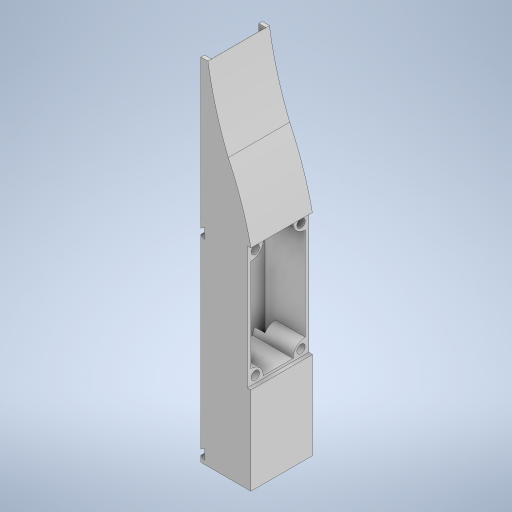
# Autodesk Inventor part: case_ver4
Saved by Autodesk Inventor 2024 (Build 280153000, 153)
## iProperties
Created: 2023-11-10
Part Number: case_ver4
Material: 一般
Document SubType Name: Modeling
Designer: Kota Taga
Density: 1 g/cm^3
Appearance: 既定
Author: Kota Taga
## iProperties of the stored document case_3D プリント.ipt
Created: 2023-11-10
Part Number: case_3D プリント
Material: 一般
Document SubType Name: Modeling
Designer: Kota Taga
Density: 1 g/cm^3
Appearance: 既定
Author: Kota Taga
Autodesk Inventor part; units mm, degrees
ref_plane "YZ Plane" through (0, 0, 0) normal (1, 0, 0) x (0, 1, 0)
ref_plane "XZ Plane" through (0, 0, 0) normal (0, 1, 0) x (-1, 0, 0)
ref_plane "XY Plane" through (0, 0, 0) normal (0, 0, 1) x (1, 0, 0)
sketch "スケッチ1" plane through (0, 0, 0) normal (0, 1, 0) x (-1, 0, 0)
  line L0 (10.25, 18.25) -> (-10.25, 18.25)
  line L1 (-10.25, 18.25) -> (-10.25, -18.25)
  line L2 (-10.25, -18.25) -> (10.25, -18.25)
  line L3 (10.25, -18.25) -> (10.25, 18.25)
  line L4 (23.2518, 0) -> (-17.5836, 0) projected
  line L5 (0, -27.65) -> (0, 27.65) projected
  line L6 (11.75, 19.75) -> (-11.75, 19.75)
  line L7 (-11.75, 19.75) -> (-11.75, -19.75)
  line L8 (-11.75, -19.75) -> (11.75, -19.75)
  line L9 (11.75, -19.75) -> (11.75, 19.75)
  line L10 (17.4182, 0.0611) -> (-9.1818, 0.0611)
  point P0 (0, 0)
  dimension "d0" = 36.5
  dimension "d1" = 20.5
  dimension "d2" = 1.5
  constraints: 18 end point, 5 parallel, 2 perpendicular, 1 horizontal, 5 other
  measures "d0" distance of L2.end L0.start
  measures "d1" distance of L0.start L0.end
  measures "d2" distance between parallel lines of L3 L9
extrude "押し出し1" add sketch "スケッチ1" along normal blind 70 contours L0 L5 L6 L9 L10 L3 | L0 L1 L4 L7 L6 L5 | L10 L9 L4 L3 | L4 L9 L8 L5 L2 L3 | L1 L2 L5 L8 L7 L4
sketch "スケッチ2" plane through (-11.75, 0, -19.75) normal (-1, 0, 0) x (0, 0, 1)
  line L0 (38, 0) -> (1.5, 0) projected
  line L1 (0, 70) -> (1.75, 70)
  line L2 (1.75, 70) -> (1.75, 0)
  line L3 (1.75, 0) -> (0, 0)
  line L4 (0, 0) -> (0, 70)
  line L5 (39.5, 0) -> (39.5, 70) projected
  line L6 (39.5, 70) -> (37.75, 70)
  line L7 (37.75, 70) -> (37.75, 0)
  line L8 (37.75, 0) -> (39.5, 0)
  line L9 (39.5, 0) -> (39.5, 70)
  point P0 (19.75, 0)
  point P1 (1.5, 0)
  dimension "d5" = 1.75
  dimension "d6" = 1.75
  constraints: 16 end point, 4 parallel, 2 horizontal, 2 perpendicular, 2 point on line
  measures "d5" distance of L2.end L3.end
  measures "d6" distance of L8.end L7.end
extrude "押し出し2" add sketch "スケッチ2" along normal blind 19
sketch "スケッチ3" plane through (11.75, 0, 19.75) normal (1, 0, 0) x (0, 0, -1)
  line L0 (0, 70) -> (39.5, 70) projected
  line L1 (39.5, 0) -> (39.5, 70) projected
  line L2 (0, 70) -> (39.5, 70)
  line L3 (39.5, 70) -> (39.5, 0)
  line L4 (39.5, 0) -> (0, 0)
  line L5 (0, 0) -> (0, 70)
  point P0 (19.75, 0)
  constraints: 8 end point, 2 parallel, 1 horizontal, 1 perpendicular
extrude "押し出し3" cut sketch "スケッチ3" against normal up to surface (1.5 mm away)
sketch "スケッチ4" plane through (10.25, 0, 18.25) normal (1, 0, 0) x (0, 0, -1)
  line L0 (-1.5, 70) -> (0, 70) projected
  line L1 (0, 0) -> (0, 70) projected
  line L2 (-1.5, 70) -> (0, 70)
  line L3 (0, 70) -> (0, 0)
  line L4 (0, 0) -> (-1.5, 0)
  line L5 (-1.5, 0) -> (-1.5, 70)
  line L6 (38, 70) -> (38, 0) projected
  line L7 (36.5, 0) -> (36.5, 70) projected
  line L8 (38, 70) -> (36.5, 70)
  line L9 (36.5, 70) -> (36.5, 0)
  line L10 (36.5, 0) -> (38, 0)
  line L11 (38, 0) -> (38, 70)
  point P0 (18.25, 0)
  constraints: 16 end point, 4 parallel, 2 horizontal, 2 perpendicular
extrude "押し出し4" add sketch "スケッチ4" along normal blind 14.5
sketch "スケッチ5" plane through (-10.25, 0, 18.25) normal (1, 0, 0) x (0, 0, -1)
  line L0 (38, 70) -> (36.5, 70) projected
  line L1 (0, 0) -> (0, 70) projected
  line L2 (36.5, 70) -> (0, 70)
  line L3 (0, 70) -> (0, 68.5)
  line L4 (0, 68.5) -> (36.5, 68.5)
  line L5 (36.5, 68.5) -> (36.5, 70)
  line L6 (0.25, 0) -> (0.25, 70) projected
  line L7 (36.5, 0) -> (36.5, 70) projected
  line L8 (0.25, 0) -> (36.5, 0)
  line L9 (36.5, 0) -> (36.5, 1.5)
  line L10 (36.5, 1.5) -> (0.25, 1.5)
  line L11 (0.25, 1.5) -> (0.25, 0)
  point P0 (18.25, 0)
  point P1 (0.25, 1.5)
  dimension "d13" = 1.5
  dimension "d14" = 1.5
  constraints: 16 end point, 4 parallel, 2 horizontal, 2 perpendicular, 2 point on line
  measures "d13" distance between parallel lines of L2 L4
  measures "d14" distance of L9.end L8.end
extrude "押し出し5" add sketch "スケッチ5" along normal up to surface (35 mm away) contours L1 L2 L6 L4 | L6 L2 L5 L4 | L10 L7 L8 L6
sketch "スケッチ6" plane through (0, 70, 0) normal (0, 1, 0) x (1, 0, 0)
  line L0 (24.75, -18) -> (24.75, 18.25) projected
  line L1 (24.75, -10) -> (14.75, -10)
  line L2 (14.75, -10) -> (14.75, 10)
  line L3 (14.75, 10) -> (24.75, 10)
  line L4 (24.75, 10) -> (24.75, -10)
  line L5 (-41.85, 0) -> (35.85, 0) projected
  line L6 (0, 27.65) -> (0, -27.65) projected
  point P0 (0, 0)
  dimension "d17" = 10
  dimension "d18" = 20
  constraints: 8 end point, 2 parallel, 1 horizontal, 1 perpendicular, 1 point on line, 1 other
  measures "d17" distance of L2.end L3.end
  measures "d18" distance of L1.end L2.end
extrude "押し出し6" cut sketch "スケッチ6" against normal up to surface (70 mm away)
sketch "スケッチ7" plane through (0, 0, 0) normal (0, -1, 0) x (1, 0, 0)
  line L0 (-10.25, 18.25) -> (-10.25, 18) projected
  line L1 (-10.25, 18) -> (24.75, 18) projected
  line L2 (-10.25, 18.25) -> (24.75, 18.25)
  line L3 (24.75, 18.25) -> (24.75, 18)
  line L4 (24.75, 18) -> (-10.25, 18)
  line L5 (-10.25, 18) -> (-10.25, 18.25)
  point P0 (0, 0)
  constraints: 8 end point, 2 parallel, 1 horizontal, 1 perpendicular
extrude "押し出し7" add sketch "スケッチ7" against normal up to surface (1.5 mm away)
sketch "スケッチ8" plane through (-10.25, 1.5, -18.25) normal (1, 0, 0) x (0, 0, -1)
  line L0 (0, 67) -> (-36.5, 67) projected
  circle A0 centre (-36.5, 67) radius 7.5
  line L1 (0, 67) -> (0, 0) projected
  circle A1 centre (0, 67) radius 7.5
  line L2 (-8.25, 0) -> (0, 0) projected
  circle A2 centre (0, 0) radius 7.5
  line L3 (-36.5, 0) -> (-36.5, 67) projected
  circle A3 centre (-36.5, 0) radius 7.5
  line L4 (-36.5, 7.5) -> (-36.5, 0)
  line L5 (-28.25, 0) -> (-36.5, 0) projected
  line L6 (-29, 0) -> (-36.5, 0)
  point P0 (-18.25, -1.5)
  point P1 (-36.5, 59.5)
  point P2 (-29, 67)
  point P3 (-7.5, 67)
  point P4 (0, 59.5)
  point P5 (0, 7.5)
  point P6 (-7.5, 0)
  dimension "d23" = 15
  dimension "d24" = 15
  dimension "d25" = 15
  dimension "d26" = 15
  constraints: 4 centre point, 4 end point, 2 coincident, 2 point on circle, 2 point on line, 1 collinear, 1 vertical
  measures "d23" diameter of A0
  measures "d24" diameter of A1
  measures "d25" diameter of A2
  measures "d26" diameter of A3
extrude "押し出し8" add sketch "スケッチ8" along normal up to surface (35 mm away) contours A0 L3 L0 | L1 A1 L0 | L1 L2 A2 | L3 A3 L5 picked at (-31.5627, 66.4437) picked at (-4.9373, 66.4437) picked at (-3.5133, 3.5133) picked at (-33.8566, 4.207)
sketch "スケッチ9" plane through (24.75, 0, 18.25) normal (1, 0, 0) x (0, 0, -1)
  circle A0 centre (2.5, 66) radius 2.4
  line L0 (-1.5, 70) -> (-1.5, 0) projected
  line L1 (8.25, 70) -> (-1.5, 70) projected
  circle A1 centre (34, 66) radius 2.4
  circle A2 centre (34, 4) radius 2.4
  circle A3 centre (2.5, 4) radius 2.4
  line L2 (8.25, 0) -> (-1.5, 0) projected
  line L3 (38, 0) -> (38, 70) projected
  line L4 (38, 0) -> (28.25, 0) projected
  line L5 (38, 70) -> (28.25, 70) projected
  point P0 (18.25, 0)
  point P1 (33.125, 0)
  dimension "d29" = 4.8
  dimension "d30" = 4
  dimension "d31" = 4
  dimension "d32" = 4
  dimension "d33" = 4
  dimension "d34" = 4.8
  dimension "d35" = 4
  dimension "d36" = 4
  dimension "d37" = 4.8
  dimension "d38" = 4
  dimension "d39" = 4
  dimension "d40" = 4.8
  constraints: 4 centre point, 1 midpoint
  measures "d29" diameter of A0
  measures "d30" distance from line of L0 A0.centre
  measures "d31" distance from line of L1 A0.centre
  measures "d32" distance from line of L2 A3.centre
  measures "d33" distance from line of L0 A3.centre
  measures "d34" diameter of A3
  measures "d35" distance from line of L3 A2.centre
  measures "d36" vertical distance of point (33.125, 0) A2.centre
  measures "d37" diameter of A2
  measures "d38" distance from line of L5 A1.centre
  measures "d39" distance from line of L3 A1.centre
  measures "d40" diameter of A1
extrude "押し出し9" cut sketch "スケッチ9" against normal blind 5
sketch "スケッチ10" plane through (0, 0, 0) normal (0, -1, 0) x (1, 0, 0)
  line L0 (14.75, 10) -> (24.75, 10) projected
  line L1 (24.75, -10) -> (14.75, -10) projected
  line L2 (24.75, 10) -> (14.75, 10)
  line L3 (14.75, 10) -> (14.75, -10)
  line L4 (14.75, -10) -> (24.75, -10)
  line L5 (24.75, -10) -> (24.75, 10)
  circle A0 centre (24.75, 0) radius 4
  point P0 (0, 0)
  point P1 (24.75, -4)
  point P2 (24.75, 4)
  dimension "d43" = 8
  constraints: 8 end point, 2 parallel, 1 centre point, 1 horizontal, 1 midpoint, 1 perpendicular
  measures "d43" diameter of A0
extrude "押し出し10" add sketch "スケッチ10" against normal up to surface (1.5 mm away) contours L0 L5 A0 L1 L3
sketch "スケッチ11" plane through (24.75, 0, 18.25) normal (1, 0, 0) x (0, 0, -1)
  line L0 (-1.5, 70) -> (-1.5, 0) projected
  line L1 (38, 0) -> (38, 70) projected
  line L2 (-1.5, 70) -> (38, 70)
  line L3 (38, 70) -> (38, 0)
  line L4 (38, 0) -> (-1.5, 0)
  line L5 (-1.5, 0) -> (-1.5, 70)
  point P0 (18.25, 0)
  point P1 (-1.5, 0)
  constraints: 8 end point, 2 parallel, 1 horizontal, 1 perpendicular
extrude "押し出し11" cut sketch "スケッチ11" against normal blind 10
sketch "スケッチ13" plane through (-30.75, 0, -19.75) normal (0, 0, -1) x (-1, 0, 0)
  arc A0 (-33.4976, 96.3635) -> (-19, 122.148) centre (-76.3491, 137.4253) ccw projected
  line L0 (-19, 122.148) -> (-22.9342, 122.148)
  line L1 (-22.9342, 122.148) -> (-22.9342, 137.4253)
  line L2 (-22.9342, 137.4253) -> (-19, 137.4253)
  line L3 (-19, 137.4253) -> (-19, 122.148)
  point P0 (-30.75, 0)
  constraints: 8 end point, 2 parallel, 1 horizontal, 1 perpendicular
extrude "押し出し13" cut sketch "スケッチ13" against normal up to surface (39.5 mm away)
sketch "スケッチ14" plane through (-30.75, 0, 19.75) normal (0, 0, 1) x (1, 0, 0)
  arc A0 (19, 122.148) -> (33.4976, 96.3635) centre (76.3491, 137.4253) ccw projected
  line L0 (19, 122.148) -> (19, 70)
  line L1 (45.5, 70) -> (0, 70) projected
  line L2 (19, 70) -> (43.4941, 70)
  arc A1 (43.4941, 70) -> (33.4976, 96.3635) centre (-6.67, 66.0559) ccw projected
  arc A2 (43.4941, 70) -> (33.4976, 96.3635) centre (-6.67, 66.0559) ccw
  arc A3 (19, 122.148) -> (33.4976, 96.3635) centre (76.3491, 137.4253) ccw
  point P0 (30.75, 0)
  constraints: 4 end point, 4 point on circle, 2 centre point, 2 concentric, 1 horizontal, 1 point on line, 1 vertical
extrude "押し出し14" add sketch "スケッチ14" against normal blind 2
mirror "ミラー1" about plane through (0, 0, 0) normal (0, 0, 1) of "押し出し14"
sketch "スケッチ15" plane through (0, 70, 0) normal (0, 1, 0) x (1, 0, 0)
  line L0 (-11.75, 17.75) -> (-11.75, -17.75) projected
  line L1 (12.7441, 17.75) -> (-11.75, 17.75) projected
  line L2 (-11.75, -17.75) -> (0.497, -17.75)
  line L3 (0.497, -17.75) -> (0.497, 17.75)
  line L4 (0.497, 17.75) -> (-11.75, 17.75)
  line L5 (-11.75, 17.75) -> (-11.75, -17.75)
  point P0 (0, 0)
  constraints: 8 end point, 2 parallel, 1 horizontal, 1 midpoint, 1 perpendicular
extrude "押し出し15" cut sketch "スケッチ15" against normal blind 2
sketch "スケッチ17" plane through (0, 70, 0) normal (0, 1, 0) x (1, 0, 0)
  line L0 (-30.75, -19.75) -> (-30.75, -18) projected
  line L1 (-11.75, -18) -> (-30.75, -18) projected
  line L2 (-30.75, -19.75) -> (-11.75, -19.75)
  line L3 (-11.75, -19.75) -> (-11.75, -18)
  line L4 (-11.75, -18) -> (-30.75, -18)
  line L5 (-30.75, -18) -> (-30.75, -19.75)
  line L6 (-11.75, 19.75) -> (-30.75, 19.75) projected
  line L7 (-11.75, 18) -> (-30.75, 18) projected
  line L8 (-30.75, 19.75) -> (-11.75, 19.75)
  line L9 (-11.75, 19.75) -> (-11.75, 18)
  line L10 (-11.75, 18) -> (-30.75, 18)
  line L11 (-30.75, 18) -> (-30.75, 19.75)
  point P0 (0, 0)
  constraints: 16 end point, 4 parallel, 2 horizontal, 2 perpendicular
extrude "押し出し17" [suppressed]
sketch "スケッチ18" plane through (-30.75, 0, 19.75) normal (0, 0, 1) x (1, 0, 0)
  line L0 (0, 0) -> (0, 122.148) projected
  line L1 (45.5, 0) -> (45.5, 70) projected
  line L2 (0, 0) -> (45.5, 0)
  line L3 (45.5, 0) -> (45.5, 70)
  line L4 (45.5, 70) -> (0, 70)
  line L5 (0, 70) -> (0, 0)
  line L6 (0, 70) -> (0, 122.148)
  line L7 (19, 68) -> (19, 122.148) projected
  line L8 (0, 122.148) -> (21.0723, 122.148) projected
  line L9 (0, 122.148) -> (19.5705, 122.148)
  arc A0 (21.4839, 120.7302) -> (19.5705, 122.148) centre (19.5705, 120.148) ccw projected
  arc A1 (21.4839, 120.7302) -> (19.5705, 122.148) centre (19.5705, 120.148) ccw
  arc A2 (45.5, 70) -> (35.0218, 97.6639) centre (-6.67, 66.0559) ccw projected
  arc A3 (21.4839, 120.7302) -> (35.0218, 97.6639) centre (76.3491, 137.4253) ccw
  arc A4 (45.5, 70) -> (35.0218, 97.6639) centre (-6.67, 66.0559) ccw
  point P0 (30.75, 0)
  constraints: 12 end point, 6 point on circle, 3 centre point, 3 parallel, 2 tangent, 1 collinear, 1 horizontal, 1 perpendicular
extrude "押し出し18" add sketch "スケッチ18" along normal blind 1
sketch "スケッチ19" plane through (14.75, 0, -19.75) normal (0, 0, -1) x (-1, 0, 0)
  arc A0 (10.4782, 97.6639) -> (0, 70) centre (52.17, 66.0559) ccw projected
  line L0 (45.5, 122.148) -> (45.5, 0) projected
  line L1 (0, 70) -> (45.5, 70)
  line L2 (45.5, 70) -> (45.5, 0)
  line L3 (45.5, 0) -> (0, 0)
  line L4 (0, 0) -> (0, 70)
  line L5 (45.5, 70) -> (45.5, 122.148)
  line L6 (26.5, 122.148) -> (45.5, 122.148) projected
  line L7 (45.5, 122.148) -> (26.5, 122.148)
  arc A1 (12.0024, 96.3635) -> (26.5, 122.148) centre (-30.8491, 137.4253) ccw projected
  line L8 (24.4277, 122.148) -> (26.5, 122.148) projected
  line L9 (26.5, 122.148) -> (25.9295, 122.148)
  arc A2 (25.9295, 122.148) -> (24.0161, 120.7302) centre (25.9295, 120.148) ccw projected
  arc A3 (25.9295, 122.148) -> (24.0161, 120.7302) centre (25.9295, 120.148) ccw
  arc A4 (10.4782, 97.6639) -> (24.0161, 120.7302) centre (-30.8491, 137.4253) ccw
  arc A5 (10.4782, 97.6639) -> (0, 70) centre (52.17, 66.0559) ccw
  point P0 (14.75, 0)
  constraints: 14 end point, 6 point on circle, 3 centre point, 3 collinear, 2 parallel, 1 concentric, 1 horizontal, 1 perpendicular
extrude "押し出し19" add sketch "スケッチ19" along normal blind 1
sketch "スケッチ20" plane through (0, 0, 0) normal (0, -1, 0) x (1, 0, 0)
  line L0 (-11.75, -18) -> (-11.75, -17.75) projected
  line L1 (-30.75, -19.75) -> (-30.75, -20.75) projected
  line L2 (-11.75, -18) -> (-30.75, -18)
  line L3 (-30.75, -18) -> (-30.75, -18.5)
  line L4 (-30.75, -18.5) -> (-11.75, -18.5)
  line L5 (-11.75, -18.5) -> (-11.75, -18)
  line L6 (-11.75, 18) -> (-30.75, 18) projected
  line L7 (-11.75, 18) -> (-30.75, 18)
  line L8 (-30.75, 18) -> (-30.75, 18.5)
  line L9 (-30.75, 18.5) -> (-11.75, 18.5)
  line L10 (-11.75, 18.5) -> (-11.75, 18)
  point P0 (0, 0)
  dimension "d69" = 0.5
  dimension "d70" = 0.5
  constraints: 16 end point, 4 parallel, 2 horizontal, 2 perpendicular, 2 point on line
  measures "d69" distance of L3.end L2.end
  measures "d70" distance of L7.end L8.end
extrude "押し出し20" [suppressed]
sketch "スケッチ23" plane through (14.75, 0, 20.75) normal (1, 0, 0) x (0, 0, -1)
  line L0 (41.5, 70) -> (0, 70) projected
  line L1 (41.5, 0) -> (41.5, 122.148) projected
  line L2 (0, 70) -> (41.5, 70)
  line L3 (41.5, 70) -> (41.5, 0)
  line L4 (41.5, 0) -> (0, 0)
  line L5 (0, 0) -> (0, 70)
  line L6 (31.5, 68.5) -> (10, 68.5) projected
  line L7 (10, 68.5) -> (31.5, 68.5)
  line L8 (10, 1.5) -> (31.5, 1.5) projected
  line L9 (10, 1.5) -> (31.5, 1.5)
  arc A0 (39, 9) -> (31.5, 1.5) centre (39, 1.5) ccw projected
  line L10 (39, 9) -> (39, 61.074)
  arc A1 (2.5, 61) -> (9.9833, 68) centre (2.5, 68.5) ccw projected
  line L11 (2.5, 61) -> (2.5, 9)
  arc A2 (10, 1.5) -> (2.5, 9) centre (2.5, 1.5) ccw
  line L12 (31.5, 1.5) -> (41.5, 1.5) projected
  arc A3 (39, 9) -> (31.5, 1.5) centre (39, 1.5) ccw
  arc A4 (31.5, 68.5) -> (31.5167, 68) centre (39, 68.5) ccw projected
  arc A5 (31.5, 68.5) -> (39, 61) centre (39, 68.5) ccw
  arc A6 (31.5, 68.5) -> (39, 61) centre (39, 68.5) ccw projected
  arc A7 (9.9833, 68) -> (10, 68.5) centre (2.5, 68.5) ccw projected
  arc A8 (2.5, 61) -> (10, 68.5) centre (2.5, 68.5) ccw
  point P0 (20.75, 0)
  point P1 (31.5167, 68)
  constraints: 16 end point, 9 point on circle, 4 centre point, 4 concentric, 4 parallel, 2 collinear, 1 horizontal, 1 perpendicular, 1 point on line
extrude "押し出し23" cut sketch "スケッチ23" against normal blind 2
sketch "スケッチ25" plane through (-11.75, 68, 17.75) normal (-1, 0, 0) x (0, 0, 1)
  line L0 (-35.5, 54.148) -> (0, 54.148) projected
  line L1 (-12.75, 49.148) -> (-22.75, 49.148) projected
  line L2 (-12.75, 54.148) -> (-22.75, 54.148)
  line L3 (-22.75, 54.148) -> (-22.75, 49.148)
  line L4 (-22.75, 49.148) -> (-12.75, 49.148)
  line L5 (-12.75, 49.148) -> (-12.75, 54.148)
  point P0 (-17.75, -68)
  constraints: 8 end point, 2 parallel, 1 horizontal, 1 perpendicular
extrude "押し出し25" cut sketch "スケッチ25" against normal blind 5
sketch "スケッチ27" plane through (0, 68, 0) normal (0, 1, 0) x (1, 0, 0)
  line L0 (-11.75, 17.75) -> (0.497, 17.75) projected
  line L1 (0.497, 17.75) -> (-11.75, 17.75)
  line L2 (-11.75, 17.75) -> (-11.75, -17.75)
  line L3 (-11.75, -17.75) -> (0.497, -17.75)
  line L4 (0.497, -17.75) -> (0.497, 17.75)
  line L5 (0.497, 10.7667) -> (-10.25, 10.7667) projected
  line L6 (0.497, 10.7667) -> (-10.25, 10.7667)
  line L7 (-10.25, -10.7667) -> (0.497, -10.7667) projected
  line L8 (-10.25, 10.7667) -> (-10.25, -10.7667)
  line L9 (0.497, -10.75) -> (0.497, 10.75) projected
  line L10 (-10.25, -10.7667) -> (0.497, -10.75)
  point P0 (0, 0)
  constraints: 14 end point, 3 equal length, 2 perpendicular, 1 horizontal
extrude "押し出し27" add sketch "スケッチ27" along normal up to surface (2 mm away) contours L0 L4 L5 L8 L7 L3 L2
sketch "スケッチ29" plane through (0, 0, 0) normal (0, -1, 0) x (1, 0, 0)
  line L0 (-30.75, 20.75) -> (12.75, 20.75) projected
  line L1 (12.75, -20.75) -> (-30.75, -20.75)
  line L2 (-30.75, -20.75) -> (-30.75, 20.75)
  line L3 (-30.75, 20.75) -> (12.75, 20.75)
  line L4 (12.75, 20.75) -> (12.75, -20.75)
  line L5 (-11.75, -18.5) -> (-30.75, -18.5) projected
  line L6 (-30.75, 18.5) -> (-11.75, 18.5) projected
  line L7 (-11.75, -18.5) -> (-30.75, -18.5)
  line L8 (-30.75, -18.5) -> (-30.75, 18.5)
  line L9 (-30.75, 18.5) -> (-11.75, 18.5)
  line L10 (-11.75, 18.5) -> (-11.75, -18.5)
  point P0 (0, 0)
  point P1 (12.75, 20.75)
  constraints: 16 end point, 4 parallel, 2 horizontal, 2 perpendicular
extrude "押し出し28" add sketch "スケッチ29" along normal blind 50 contours L0 L4 L1 L2 L5 L10 L6
sketch "スケッチ30" plane through (12.75, 0, 20.75) normal (1, 0, 0) x (0, 0, -1)
  line L0 (41.5, 70) -> (41.5, -50) projected
  line L1 (0, 0) -> (41.5, 0)
  line L2 (41.5, 0) -> (41.5, -50)
  line L3 (41.5, -50) -> (0, -50)
  line L4 (0, -50) -> (0, 0)
  line L5 (10, 1.5) -> (31.5, 1.5) projected
  point P0 (20.75, 0)
  dimension "d105" = 1.5
  constraints: 8 end point, 2 parallel, 1 horizontal, 1 perpendicular
  measures "d105" distance between parallel lines of L1 L5
extrude "押し出し29" add sketch "スケッチ30" along normal blind 2
sketch "スケッチ31" plane through (12.75, 0, 20.75) normal (1, 0, 0) x (0, 0, -1)
  line L0 (0, 0) -> (0, 70) projected
  line L1 (41.5, 122.148) -> (41.5, -50) projected
  line L2 (0, 70) -> (41.5, 70)
  line L3 (41.5, 70) -> (41.5, 122.148)
  line L4 (41.5, 122.148) -> (0, 122.148)
  line L5 (0, 122.148) -> (0, 70)
  point P0 (20.75, 0)
  constraints: 8 end point, 2 parallel, 1 horizontal, 1 perpendicular
extrude "押し出し30" cut sketch "スケッチ31" along normal mid plane 100
sketch "スケッチ32" plane through (14.75, 0, -20.75) normal (0, 0, -1) x (-1, 0, 0)
  line L0 (2, 70) -> (2, 0) projected
  line L1 (2, 70) -> (45.5, 70)
  line L2 (45.5, 70) -> (45.5, 150)
  line L3 (45.5, 150) -> (2, 150)
  line L4 (2, 150) -> (2, 70)
  line L5 (43.5, 150) -> (43.5, 70)
  line L6 (26.5, 70) -> (26.5, 0) projected
  line L7 (26.5, 70) -> (26.5, 150)
  arc A0 (14.75, 107.3844) -> (26.5, 150) centre (-163.08, 179.3435) ccw
  arc A1 (14.75, 107.3844) -> (2, 70) centre (176.3972, 31.388) ccw
  point P0 (14.75, 0)
  dimension "d110" = 80
  dimension "d111" = 2
  constraints: 12 end point, 5 point on circle, 3 perpendicular, 3 point on line, 2 centre point, 2 parallel, 1 horizontal
  measures "d110" distance of L2.end L1.end
  measures "d111" distance between parallel lines of L2 L5
extrude "押し出し31" add sketch "スケッチ32" against normal up to surface (41.5 mm away) contours A1 A0 L7 L1 | L7 L3 L5 L1 | L5 L3 L2 L1
sketch "スケッチ33" plane through (-30.75, 70, -18) normal (0, -1, 0) x (1, 0, 0)
  line L0 (0, 0) -> (0, 36) projected
  line L1 (0, 0) -> (19, 0)
  line L2 (19, 0) -> (19, 36)
  line L3 (19, 36) -> (0, 36)
  line L4 (0, 36) -> (0, 0)
  point P0 (30.75, 18)
  constraints: 8 end point, 2 parallel, 1 horizontal, 1 perpendicular
extrude "押し出し32" cut sketch "スケッチ33" against normal up to surface (80 mm away)
sketch "スケッチ34" plane through (14.75, 0, -20.75) normal (0, 0, -1) x (-1, 0, 0)
  line L0 (244.2926, 0) -> (-230.9754, 0) projected
  line L1 (14.75, -95.8687) -> (14.75, 225.2121) projected
  arc A0 (14.75, 107.3844) -> (26.5, 150) centre (-163.08, 179.3435) ccw projected
  line L2 (26.5, 0) -> (26.5, 150) projected
  arc A1 (14.75, 107.3844) -> (26.5, 150) centre (-163.08, 179.3435) ccw
  arc A2 (14.75, 107.3844) -> (2, 70) centre (176.3972, 31.388) ccw projected
  arc A3 (14.75, 107.3844) -> (2, 70) centre (176.3972, 31.388) ccw
  arc A4 (12.896, 108.1346) -> (24.5235, 150.3059) centre (-163.08, 179.3435) ccw
  line L3 (2, 70) -> (0, 70)
  arc A5 (12.896, 108.1346) -> (0, 70) centre (169.661, 33.8733) ccw
  line L4 (26.5, 150) -> (45.5, 150) projected
  line L5 (26.5, 150) -> (24.4759, 150)
  point P0 (14.75, 0)
  dimension "d116" = 2
  constraints: 9 point on circle, 4 centre point, 4 end point, 1 collinear, 1 horizontal
  measures "d116" radial gap between concentric circles of A0 A4
extrude "押し出し33" add sketch "スケッチ34" against normal up to surface (41.5 mm away) contours A0 L1 A4 L5 | A2 L3 A5 A4 L1
ref_plane "作業平面1" through (-30.75, 0, 0) normal (0, 0, 1) x (1, 0, 0)
sketch "スケッチ36" plane through (-30.75, 0, 0) normal (0, 0, 1) x (1, 0, 0)
  line L0 (31.247, 68) -> (31.247, 70) projected
  line L1 (31.247, 70) -> (20.5, 70)
  line L2 (20.5, 70) -> (20.5, 90)
  line L3 (20.5, 90) -> (31.247, 90)
  line L4 (31.247, 90) -> (31.247, 70)
  line L5 (19, 0) -> (19, 150) projected
  line L6 (20.5, 90) -> (19, 90)
  line L7 (19, 90) -> (19, 70)
  line L8 (19, 70) -> (20.5, 70)
  line L9 (20.5, 70) -> (20.5, 90)
  point P0 (30.75, 0)
  dimension "d121" = 20
  constraints: 16 end point, 4 parallel, 2 horizontal, 2 perpendicular, 2 point on line
  measures "d121" distance of L1.end L2.end
extrude "押し出し34" cut sketch "スケッチ36" along normal up to surface (10.7667 mm away)
mirror "ミラー2" about plane through (-30.75, 0, 0) normal (0, 0, 1) of "押し出し34"
sketch "スケッチ37" plane through (-11.75, -50, -18.5) normal (-1, 0, 0) x (0, 0, 1)
  line L0 (29.2667, 140) -> (7.7333, 140) projected
  line L1 (-2.25, 200) -> (39.25, 200) projected
  line L2 (7.7333, 140) -> (29.3064, 140)
  line L3 (29.3064, 140) -> (29.3064, 200)
  line L4 (29.3064, 200) -> (7.7333, 200)
  line L5 (7.7333, 200) -> (7.7333, 140)
  point P0 (18.5, 50)
  constraints: 8 end point, 2 parallel, 1 horizontal, 1 perpendicular, 1 point on line
extrude "押し出し35" cut sketch "スケッチ37" against normal blind 2
sketch "スケッチ38" plane through (-30.75, 0, -19.75) normal (-1, 0, 0) x (0, 0, 1)
  line L0 (1.25, 0) -> (1.25, -50) projected
  line L1 (-1, 150) -> (40.5, 150) projected
  line L2 (1.25, 0) -> (38.25, 0)
  line L3 (38.25, 0) -> (38.25, 150)
  line L4 (38.25, 150) -> (1.25, 150)
  line L5 (1.25, 150) -> (1.25, 0)
  point P0 (19.75, 0)
  dimension "d126" = 37
  constraints: 8 end point, 2 parallel, 1 horizontal, 1 perpendicular, 1 point on line
  measures "d126" distance of L4.end L3.end
extrude "押し出し36" cut sketch "スケッチ38" against normal up to surface (19 mm away)
sketch "スケッチ39" plane through (-30.75, 0, -19.75) normal (-1, 0, 0) x (0, 0, 1)
  line L0 (0.75, -10) -> (38.75, -10)
  line L1 (38.75, -10) -> (38.75, -50)
  line L2 (38.75, -50) -> (0.75, -50)
  line L3 (0.75, -50) -> (0.75, -10)
  line L4 (38.25, -50) -> (1.25, -50) projected
  line L5 (19.75, -90) -> (19.75, 190) projected
  line L6 (-9.3, 0) -> (48.8, 0) projected
  point P0 (19.75, 0)
  dimension "d129" = 38
  dimension "d130" = 40
  dimension "d131" = 0
  constraints: 8 end point, 2 parallel, 1 horizontal, 1 perpendicular, 1 other
  measures "d129" distance of L0.start L0.end
  measures "d130" distance of L0.end L1.end
  measures "d131" distance between parallel lines of L2 L4
extrude "押し出し37" cut sketch "スケッチ39" against normal up to surface (19 mm away)
sketch "スケッチ40" plane through (-30.75, 0, -19.75) normal (-1, 0, 0) x (0, 0, 1)
  line L0 (1.25, -10) -> (1.25, 150) projected
  line L1 (1.25, 150) -> (8.9833, 150) projected
  line L2 (1.25, -10) -> (2.25, -10)
  line L3 (2.25, -10) -> (2.25, 150)
  line L4 (2.25, 150) -> (1.25, 150)
  line L5 (1.25, 150) -> (1.25, -10)
  line L6 (38.25, 150) -> (38.25, -10) projected
  line L7 (38.25, 150) -> (37.25, 150)
  line L8 (37.25, 150) -> (37.25, -10)
  line L9 (37.25, -10) -> (38.25, -10)
  line L10 (38.25, -10) -> (38.25, 150)
  line L11 (19.75, -90) -> (19.75, 190) projected
  point P0 (19.75, 0)
  dimension "d134" = 35
  constraints: 16 end point, 4 parallel, 2 horizontal, 2 perpendicular, 1 point on line, 1 other
  measures "d134" distance between parallel lines of L8 L3
extrude "押し出し38" add sketch "スケッチ40" against normal up to surface (19 mm away)
sketch "スケッチ41" plane through (-30.75, 0, -19.75) normal (-1, 0, 0) x (0, 0, 1)
  line L0 (37.25, 150) -> (37.25, -10) projected
  line L1 (40.5, 150) -> (40.5, -50) projected
  line L2 (37.25, 150) -> (40.5, 150)
  line L3 (40.5, 150) -> (40.5, -10.0917)
  line L4 (40.5, -10.0917) -> (37.25, -10.0917)
  line L5 (37.25, -10.0917) -> (37.25, 150)
  line L6 (40.5, -50) -> (38.75, -50) projected
  line L7 (38.75, -50) -> (40.5, -50)
  line L8 (40.5, -50) -> (40.5, -10.0917)
  line L9 (40.5, -10.0917) -> (38.75, -10.0917)
  line L10 (38.75, -10.0917) -> (38.75, -50)
  point P0 (19.75, 0)
  constraints: 16 end point, 4 parallel, 2 horizontal, 2 perpendicular, 1 point on line
extrude "押し出し39" add sketch "スケッチ41" along normal blind 2
ref_plane "作業平面2" through (-10.25, 9, -18.25) normal (0, 1, 0) x (-1, 0, 0)
mirror "ミラー3" about plane through (-30.75, 0, 0) normal (0, 0, 1) of "押し出し39"
sketch "スケッチ45" plane through (-9.7259, 150, 20.75) normal (0, 1, 0) x (1, 0, 0)
  line L0 (0, 0) -> (-23.0241, 0) projected
  line L1 (0, 41.5) -> (0, 0) projected
  line L2 (-23.0241, 0) -> (0, 0)
  line L3 (0, 0) -> (0, 3.25)
  line L4 (0, 3.25) -> (-23.0241, 3.25)
  line L5 (-23.0241, 3.25) -> (-23.0241, 0)
  line L6 (-23.0241, 41.5) -> (0, 41.5) projected
  line L7 (-0.5241, 38.25) -> (1.4759, 38.25) projected
  line L8 (-23.0241, 41.5) -> (0, 41.5)
  line L9 (0, 41.5) -> (0, 38.25)
  line L10 (0, 38.25) -> (-23.0241, 38.25)
  line L11 (-23.0241, 38.25) -> (-23.0241, 41.5)
  line L12 (0, 0) -> (11.5799, 0) projected
  line L13 (0, 0) -> (27.7605, 0)
  line L14 (27.7605, 0) -> (27.7605, 3.25)
  line L15 (27.7605, 3.25) -> (0, 3.25)
  line L16 (0, 3.25) -> (0, 0)
  line L17 (0, 41.5) -> (28.7507, 41.5)
  line L18 (28.7507, 41.5) -> (28.7507, 38.25)
  line L19 (28.7507, 38.25) -> (0, 38.25)
  line L20 (0, 38.25) -> (0, 41.5)
  point P0 (9.7259, 20.75)
  point P1 (0, 3.25)
  dimension "d147" = 3.25
  constraints: 32 end point, 8 parallel, 4 horizontal, 4 perpendicular, 3 point on line
  measures "d147" distance of L3.end L2.end
extrude "押し出し42" cut sketch "スケッチ45" against normal up to surface (200 mm away)
sketch "スケッチ46" plane through (12.75, 0, 20.75) normal (1, 0, 0) x (0, 0, -1)
  line L0 (10, 68.5) -> (31.5, 68.5) projected
  line L1 (38.25, 150) -> (38.25, -50) projected
  line L2 (31.5, 68.5) -> (38.25, 68.5)
  line L3 (38.25, 68.5) -> (38.25, 59.4183)
  line L4 (38.25, 59.4183) -> (31.5, 59.4183)
  line L5 (31.5, 59.4183) -> (31.5, 68.5)
  line L6 (3.25, -50) -> (3.25, 150) projected
  line L7 (9.9833, 68.5) -> (3.25, 68.5)
  line L8 (3.25, 68.5) -> (3.25, 58.3642)
  line L9 (3.25, 58.3642) -> (9.9833, 58.3642)
  line L10 (9.9833, 58.3642) -> (9.9833, 68.5)
  arc A0 (38.25, 8.9624) -> (31.5, 1.5) centre (39, 1.5) ccw projected
  line L11 (31.5, 1.5) -> (38.25, 1.5)
  line L12 (38.25, 1.5) -> (38.25, 11.6398)
  line L13 (38.25, 11.6398) -> (31.5, 11.6398)
  line L14 (31.5, 11.6398) -> (31.5, 1.5)
  line L15 (9.9833, 1.5) -> (3.25, 1.5)
  line L16 (3.25, 1.5) -> (3.25, 11.6398)
  line L17 (3.25, 11.6398) -> (9.9833, 11.6398)
  line L18 (9.9833, 11.6398) -> (9.9833, 1.5)
  point P0 (20.75, 0)
  constraints: 32 end point, 8 parallel, 8 point on line, 4 horizontal, 4 perpendicular
extrude "押し出し43" cut sketch "スケッチ46" against normal up to surface (23 mm away) contours L1 L4 L5 L2 | L1 L11 A0 | L6 L17 L18 L15 | L6 L7 L10 L9
sketch "スケッチ47" plane through (-10.25, 70, 10.7667) normal (1, 0, 0) x (0, 0, -1)
  line L0 (0.0167, -1.5) -> (28.2667, -1.5) projected
  line L1 (28.2667, -68.5) -> (0.0167, -68.5) projected
  line L2 (28.2667, -1.5) -> (26.2667, -1.5)
  line L3 (26.2667, -1.5) -> (26.2667, -68.5)
  line L4 (26.2667, -68.5) -> (28.2667, -68.5)
  line L5 (28.2667, -68.5) -> (28.2667, -1.5)
  line L6 (-6.7333, -68.5) -> (-4.7333, -68.5)
  line L7 (-4.7333, -68.5) -> (-4.7333, -1.5)
  line L8 (-4.7333, -1.5) -> (-6.7333, -1.5)
  line L9 (-6.7333, -1.5) -> (-6.7333, -68.5)
  point P0 (10.7667, -70)
  dimension "d152" = 2
  dimension "d153" = 2
  constraints: 16 end point, 4 parallel, 3 point on line, 2 horizontal, 2 perpendicular
  measures "d152" distance of L4.end L3.end
  measures "d153" distance of L8.end L7.end
extrude "押し出し44" add sketch "スケッチ47" along normal up to surface (23 mm away)
sketch "スケッチ49" plane through (12.75, 0, 20.75) normal (1, 0, 0) x (0, 0, -1)
  line L0 (9.9833, 1.5) -> (5.25, 1.5) projected
  line L1 (9.7922, 1.5) -> (10.1687, 1.5)
  line L2 (10.1687, 1.5) -> (10.1687, 2.0529)
  line L3 (10.1687, 2.0529) -> (9.7922, 2.0529)
  line L4 (9.7922, 2.0529) -> (9.7922, 1.5)
  line L5 (5.25, 68.5) -> (9.9833, 68.5) projected
  line L6 (9.3467, 68.5) -> (10.5051, 68.5)
  line L7 (10.5051, 68.5) -> (10.5051, 67.8288)
  line L8 (10.5051, 67.8288) -> (9.3467, 67.8288)
  line L9 (9.3467, 67.8288) -> (9.3467, 68.5)
  point P0 (20.75, 0)
  constraints: 16 end point, 4 parallel, 2 horizontal, 2 perpendicular, 2 point on line
extrude "押し出し45" cut sketch "スケッチ49" against normal up to surface (23 mm away)
sketch "スケッチ50" plane through (12.75, 0, 20.75) normal (1, 0, 0) x (0, 0, -1)
  line L0 (3.25, 70) -> (3.25, 0) projected
  line L1 (3.25, 0) -> (7.75, 0)
  line L2 (7.75, 0) -> (7.75, 4)
  line L3 (7.75, 4) -> (3.25, 4)
  line L4 (3.25, 4) -> (3.25, 0)
  circle A0 centre (7.75, 4) radius 2.35
  circle A1 centre (7.75, 66) radius 2.35
  circle A2 centre (33.75, 66) radius 2.35
  circle A3 centre (33.75, 4) radius 2.35
  line L5 (38.25, 70) -> (3.25, 70) projected
  line L6 (38.25, 0) -> (38.25, 70) projected
  line L7 (38.25, 0) -> (3.25, 0) projected
  line L8 (5.25, 68.5) -> (9.9833, 68.5) projected
  circle A4 centre (5.25, 68.5) radius 7
  line L9 (36.25, 1.5) -> (36.25, 68.5) projected
  circle A5 centre (36.25, 68.5) radius 7
  line L10 (5.25, 68.5) -> (5.25, 1.5) projected
  circle A6 centre (5.25, 1.5) radius 7
  circle A7 centre (36.25, 1.5) radius 7
  point P0 (20.75, 0)
  point P1 (12.0874, 0)
  point P2 (3.25, 8.2082)
  point P3 (29.4126, 0)
  point P4 (38.25, 8.2082)
  point P5 (38.25, 61.7918)
  point P6 (29.4126, 70)
  point P7 (12.0874, 70)
  point P8 (3.25, 61.7918)
  dimension "d158" = 4.5
  dimension "d159" = 4
  dimension "d160" = 4.7
  dimension "d161" = 4.5
  dimension "d162" = 4
  dimension "d163" = 4.7
  dimension "d164" = 4.5
  dimension "d165" = 4
  dimension "d166" = 4.7
  dimension "d167" = 4.5
  dimension "d168" = 4
  dimension "d169" = 4.7
  dimension "d170" = 14
  dimension "d171" = 14
  dimension "d172" = 14
  dimension "d173" = 14
  constraints: 8 centre point, 8 end point, 2 coincident, 2 parallel, 1 horizontal, 1 perpendicular
  measures "d158" distance of L3.end L2.end
  measures "d159" distance of L2.end L1.end
  measures "d160" diameter of A0
  measures "d161" distance from line of L0 A1.centre
  measures "d162" distance from line of L5 A1.centre
  measures "d163" diameter of A1
  measures "d164" distance from line of L6 A2.centre
  measures "d165" distance from line of L5 A2.centre
  measures "d166" diameter of A2
  measures "d167" distance from line of L6 A3.centre
  measures "d168" distance from line of L7 A3.centre
  measures "d169" diameter of A3
  measures "d170" diameter of A4
  measures "d171" diameter of A5
  measures "d172" diameter of A6
  measures "d173" diameter of A7
extrude "押し出し46" add sketch "スケッチ50" against normal up to surface (23 mm away) contours L3 A0 L2 L1 L0 | L0 A6 L10 L3 | L10 A6 L7 L2 A0 L3 | L0 L5 A4 | A7 L6 L7 | L5 L6 A5 picked at (3.9667, 65.9306) picked at (37.5333, 4.0694) picked at (37.5333, 65.9306)
sketch "スケッチ51" plane through (-10.25, 66, 13) normal (1, 0, 0) x (0, 0, -1)
  circle A0 centre (0, 0) radius 2.35 projected
  circle A1 centre (0, 0) radius 2.35
  circle A2 centre (26, 0) radius 2.35 projected
  circle A3 centre (26, 0) radius 2.35
  circle A4 centre (26, -62) radius 2.35 projected
  circle A5 centre (26, -62) radius 2.35
  circle A6 centre (0, -62) radius 2.35 projected
  circle A7 centre (0, -62) radius 2.35
  point P0 (13, -66)
  constraints: 4 centre point, 4 coincident
extrude "押し出し47" add sketch "スケッチ51" along normal blind 18
ref_plane "作業平面3" through (12.75, 8.5, -15.5) normal (0, 1, 0) x (-1, 0, 0)
sketch "スケッチ57" plane through (12.75, 8.5, -15.5) normal (0, 1, 0) x (-1, 0, 0)
  line L0 (23, 0) -> (23, 7) projected
  line L1 (23, 0) -> (17, 0)
  line L2 (17, 0) -> (17, 6)
  line L3 (17, 6) -> (23, 6)
  line L4 (23, 6) -> (23, 0)
  point P0 (12.75, 15.5)
  dimension "d210" = 6
  dimension "d211" = 6
  constraints: 8 end point, 2 parallel, 1 horizontal, 1 perpendicular
  measures "d210" distance of L2.end L3.end
  measures "d211" distance of L1.end L2.end
extrude "押し出し53" cut sketch "スケッチ57" against normal blind 56.5
sketch "スケッチ58" plane through (12.75, 0, -17.5) normal (0, 0, -1) x (-1, 0, 0)
  line L0 (23, -48) -> (23, 61.5) projected
  line L1 (17, 8.5) -> (17, -48) projected
  line L2 (23, -48) -> (17, -48)
  line L3 (17, -48) -> (17, -42)
  line L4 (17, -42) -> (23, -42)
  line L5 (23, -42) -> (23, -48)
  point P0 (12.75, 0)
  dimension "d214" = 6
  constraints: 8 end point, 2 parallel, 1 horizontal, 1 perpendicular, 1 point on line
  measures "d214" distance of L2.end L3.end
extrude "押し出し54" cut sketch "スケッチ58" against normal blind 5
sketch "スケッチ59" plane through (-11.75, 70, -10.7667) normal (-1, 0, 0) x (0, 0, 1)
  line L0 (-6.7333, 80) -> (-6.7333, -120) projected
  line L1 (0, 0) -> (0, 80) projected
  line L2 (-6.7333, 80) -> (0, 80)
  line L3 (0, 80) -> (0, 0)
  line L4 (0, 0) -> (-6.7333, 0)
  line L5 (-6.7333, 0) -> (-6.7333, 80)
  line L6 (28.2667, -120) -> (28.2667, 80) projected
  line L7 (21.5334, 0) -> (21.5334, 20) projected
  line L8 (28.2667, 80) -> (21.5334, 80)
  line L9 (21.5334, 80) -> (21.5334, 0)
  line L10 (21.5334, 0) -> (28.2667, 0)
  line L11 (28.2667, 0) -> (28.2667, 80)
  line L12 (28.2667, -120) -> (-6.7333, -120) projected
  line L13 (-6.7333, 0) -> (28.2667, 0)
  line L14 (28.2667, 0) -> (28.2667, -120)
  line L15 (28.2667, -120) -> (-6.7333, -120)
  line L16 (-6.7333, -120) -> (-6.7333, 0)
  point P0 (10.7667, -70)
  constraints: 24 end point, 6 parallel, 3 horizontal, 3 perpendicular
extrude "押し出し55" add sketch "スケッチ59" along normal blind 2
sketch "スケッチ62" plane through (12.75, 0, -17.5) normal (0, 0, -1) x (-1, 0, 0)
  line L0 (26.5, -50) -> (26.5, 150) projected
  line L1 (26.5, -42) -> (24.5, -42)
  line L2 (24.5, -42) -> (24.5, -48)
  line L3 (24.5, -48) -> (26.5, -48)
  line L4 (26.5, -48) -> (26.5, -42)
  line L5 (17, -42) -> (23, -42) projected
  line L6 (24.5, -42) -> (26.5, -43.5)
  line L7 (24.5, -48) -> (26.5, -46.5)
  point P0 (12.75, 0)
  point P1 (25.5, -42)
  dimension "d236" = 2
  dimension "d237" = 0
  dimension "d238" = 6
  dimension "d239" = 1.5
  dimension "d240" = 1.5
  constraints: 12 end point, 3 point on line, 2 parallel, 1 horizontal, 1 midpoint, 1 perpendicular
  measures "d236" distance of L3.end L2.end
  measures "d237" distance from line of L5 point (25.5, -42)
  measures "d238" distance of L1.end L2.end
  measures "d239" distance from line of L1 L6.end
  measures "d240" distance from line of L3 L7.end
extrude "押し出し58" cut sketch "スケッチ62" against normal up to surface (35 mm away) contours L7 L2 L6 L0
sketch "スケッチ63" plane through (12.75, 0, -17.5) normal (0, 0, -1) x (-1, 0, 0)
  line L0 (26.5, 150) -> (26.5, -43.5) projected
  line L1 (26.5, 67) -> (24.5, 67)
  line L2 (24.5, 67) -> (24.5, 61)
  line L3 (24.5, 61) -> (26.5, 61)
  line L4 (26.5, 61) -> (26.5, 67)
  line L5 (0, 70) -> (-2, 70) projected
  line L6 (24.5, 67) -> (26.5, 65.5)
  line L7 (24.5, 61) -> (26.5, 62.5)
  point P0 (12.75, 0)
  dimension "d243" = 2
  dimension "d244" = 6
  dimension "d245" = 3
  dimension "d246" = 1.5
  dimension "d247" = 1.5
  constraints: 12 end point, 3 point on line, 2 parallel, 1 horizontal, 1 perpendicular
  measures "d243" distance of L1.start L1.end
  measures "d244" distance of L1.end L2.end
  measures "d245" distance between parallel lines of L1 L5
  measures "d246" distance from line of L1 L6.end
  measures "d247" vertical distance of L2.end L7.end
extrude "押し出し59" cut sketch "スケッチ63" against normal up to surface (35 mm away) contours L0 L7 L2 L6
sketch "スケッチ64" plane through (-13.75, 70, -10.7667) normal (-1, 0, 0) x (0, 0, 1)
  line L0 (28.2667, 0) -> (-6.7333, 0) projected
  line L1 (28.2667, 80) -> (21.5334, 80) projected
  line L2 (-4.7333, 0) -> (26.2667, 0)
  line L3 (26.2667, 0) -> (26.2667, 80)
  line L4 (26.2667, 80) -> (-4.7333, 80)
  line L5 (-4.7333, 80) -> (-4.7333, 0)
  line L6 (28.2667, -4.5) -> (28.2667, 80) projected
  line L7 (-6.7333, 80) -> (-6.7333, -4.5) projected
  point P0 (10.7667, -70)
  point P1 (26.2667, 0)
  dimension "d250" = 2
  dimension "d251" = 2
  constraints: 8 end point, 2 parallel, 2 point on line, 1 horizontal, 1 perpendicular
  measures "d250" distance between parallel lines of L6 L3
  measures "d251" distance between parallel lines of L5 L7
extrude "押し出し60" cut sketch "スケッチ64" against normal up to surface (4 mm away) contours L0 L5 L4 L1 L3
ref_plane "作業平面4" through (-9.75, 70, -10.7667) normal (0, 1, 0) x (1, 0, 0)
sketch "スケッチ65" plane through (-9.75, 70, -10.7667) normal (0, 1, 0) x (1, 0, 0)
  line L0 (10.247, 4.7333) -> (-0.5, 4.7333)
  line L1 (-0.5, 4.7333) -> (-0.5, -26.2667)
  line L2 (-0.5, -26.2667) -> (10.247, -26.2667)
  line L3 (10.247, -26.2667) -> (10.247, 4.7333)
  line L4 (5.5, 6.7333) -> (-0.5, 6.7333) projected
  line L5 (24.5, -28.2667) -> (-4, -28.2667) projected
  line L6 (-0.5, -2.2667) -> (-0.5, -19.2667) projected
  line L7 (10.247, -2.2667) -> (10.247, -19.2667) projected
  point P0 (9.75, -10.7667)
  point P1 (4.8735, 4.7333)
  dimension "d255" = 2
  dimension "d256" = 2
  dimension "d257" = 0
  dimension "d258" = 0
  constraints: 8 end point, 2 parallel, 1 horizontal, 1 midpoint, 1 perpendicular
  measures "d255" distance from line of L4 point (4.874, 4.733)
  measures "d256" distance between parallel lines of L5 L2
  measures "d257" distance between parallel lines of L6 L1
  measures "d258" distance between parallel lines of L7 L3
extrude "押し出し61" cut sketch "スケッチ65" along normal mid plane 30
sketch "スケッチ66" plane through (-9.75, -50, -18.5) normal (-1, 0, 0) x (0, 0, 1)
  line L0 (7.7333, 135) -> (3, 135) projected
  line L1 (3, 135) -> (14.5, 135)
  line L2 (14.5, 135) -> (14.5, 155)
  line L3 (14.5, 155) -> (3, 155)
  line L4 (3, 155) -> (3, 135)
  line L5 (34, 120) -> (3, 120) projected
  point P0 (18.5, 50)
  dimension "d261" = 35
  dimension "d262" = 11.5
  constraints: 8 end point, 2 parallel, 1 horizontal, 1 perpendicular
  measures "d261" distance between parallel lines of L3 L5
  measures "d262" distance of L2.end L3.end
extrude "押し出し62" cut sketch "スケッチ66" against normal up to surface (10.247 mm away)
sketch "スケッチ67" plane through (-9.75, 70, -10.7667) normal (0, 1, 0) x (1, 0, 0)
  circle A0 centre (4.8735, -1.2667) radius 4
  line L0 (-4, 6.7333) -> (24.5, 6.7333) projected
  line L1 (10.247, -2.2667) -> (10.247, 4.7333) projected
  line L2 (22.5, 4.7333) -> (10.247, 4.7333) projected
  line L3 (-0.5, -2.2667) -> (-0.5, -19.2667) projected
  line L4 (10.247, 4.7333) -> (-0.5, 4.7333)
  line L5 (-0.5, 4.7333) -> (-0.5, -7.2667)
  line L6 (-0.5, -7.2667) -> (10.247, -7.2667)
  line L7 (10.247, -7.2667) -> (10.247, 4.7333)
  point P0 (9.75, -10.7667)
  dimension "d267" = 8
  dimension "d268" = 8
  dimension "d269" = 5.3735
  dimension "d270" = 12
  constraints: 8 end point, 2 parallel, 1 centre point, 1 horizontal, 1 perpendicular, 1 point on line
  measures "d267" diameter of A0
  measures "d268" distance from line of A0.centre L0
  measures "d269" distance from line of L1 A0.centre
  measures "d270" distance of L5.end L4.end
extrude "押し出し63" add sketch "スケッチ67" against normal up to surface (1.5 mm away)
sketch "スケッチ68" plane through (-9.75, -50, -18.5) normal (-1, 0, 0) x (0, 0, 1)
  line L0 (14.5, 155) -> (14.5, 140) projected
  line L1 (3, 120) -> (3, 200) projected
  line L2 (14.5, 155) -> (3, 155)
  line L3 (3, 155) -> (3, 160)
  line L4 (3, 160) -> (14.5, 160)
  line L5 (14.5, 160) -> (14.5, 155)
  point P0 (18.5, 50)
  dimension "d273" = 5
  constraints: 8 end point, 2 parallel, 1 horizontal, 1 midpoint, 1 perpendicular
  measures "d273" distance of L2.end L3.end
extrude "押し出し64" cut sketch "スケッチ68" against normal up to surface (10.247 mm away)
fillet "フィレット4" radius 10 1 edges at (0.497, 110, -9.75)
sketch "スケッチ69" plane through (-9.75, -50, -18.5) normal (-1, 0, 0) x (0, 0, 1)
  line L0 (14.5, 160) -> (14.5, 140) projected
  line L1 (34, 135) -> (29.2667, 135) projected
  line L2 (14.5, 150) -> (34, 150)
  line L3 (34, 150) -> (34, 135)
  line L4 (34, 135) -> (14.5, 135)
  line L5 (14.5, 135) -> (14.5, 150)
  point P0 (18.5, 50)
  constraints: 8 end point, 2 parallel, 1 horizontal, 1 midpoint, 1 perpendicular
extrude "押し出し65" cut sketch "スケッチ69" against normal up to surface (10.247 mm away)
sketch "スケッチ70" plane through (-9.75, -50, -18.5) normal (-1, 0, 0) x (0, 0, 1)
  line L0 (14.5, 160) -> (14.5, 150) projected
  line L1 (34, 200) -> (34, 120) projected
  line L2 (14.5, 150) -> (34, 150)
  line L3 (34, 150) -> (34, 160)
  line L4 (34, 160) -> (14.5, 160)
  line L5 (14.5, 160) -> (14.5, 150)
  point P0 (18.5, 50)
  constraints: 8 end point, 2 parallel, 1 horizontal, 1 midpoint, 1 perpendicular
extrude "押し出し66" cut sketch "スケッチ70" against normal up to surface (10.247 mm away)
fillet "フィレット5" radius 10 1 edges at (0.497, 110, 5.75)
sketch "スケッチ71" plane through (-9.75, 70, -10.7667) normal (0, 1, 0) x (1, 0, 0)
  circle A0 centre (4.8735, -1.2667) radius 4 projected
  circle A1 centre (4.8735, -1.2667) radius 4.5
  point P0 (9.75, -10.7667)
  dimension "d282" = 9
  constraints: 1 centre point, 1 coincident
  measures "d282" diameter of A1
extrude "押し出し67" cut sketch "スケッチ71" against normal up to surface (1.5 mm away) contours A0 | A1
fillet "フィレット6" radius 100 1 edges at (-9.75, 110, 0)
